Autodesk Fusion 360 part; units mm, degrees
note: some values were not read from the file. Set by a fixed rule: which sketch regions a step uses.
(part 10 of 15)
  line L7918 (197.419, -100.32) -> (197.381, -100.6)
  line L7919 (98.8127, -108.073) -> (99.0879, -108.136)
  line L7920 (197.381, -100.6) -> (197.304, -100.872)
  line L7921 (-22.9133, -112.864) -> (-22.9509, -113.144)
  line L7922 (-23.8113, -111.067) -> (-23.5867, -111.238)
  line L7923 (29.1335, -114.838) -> (28.9254, -114.669)
  line L7924 (-22.9888, -112.181) -> (-22.9293, -112.457)
  line L7925 (29.9879, -111.399) -> (30.2558, -111.384)
  line L7926 (-23.1418, -113.675) -> (-23.2913, -113.914)
  line L7927 (-23.2913, -113.914) -> (-23.4731, -114.13)
  line L7928 (30.2558, -111.384) -> (30.5232, -111.407)
  line L7929 (-23.9184, -114.476) -> (-24.1731, -114.598)
  line L7930 (-23.0276, -113.416) -> (-23.1418, -113.675)
  line L7931 (-22.9509, -113.144) -> (-23.0276, -113.416)
  line L7932 (-24.1731, -114.598) -> (-24.4425, -114.683)
  line L7933 (28.3543, -112.957) -> (28.419, -112.697)
  line L7934 (29.2333, -111.664) -> (29.4714, -111.54)
  line L7935 (29.7246, -111.451) -> (29.9879, -111.399)
  line L7936 (-24.5965, -110.763) -> (-24.3213, -110.827)
  line L7937 (32.0865, -113.669) -> (32.0137, -113.928)
  line L7938 (-24.3213, -110.827) -> (-24.0578, -110.929)
  line L7939 (28.8207, -112.005) -> (29.0149, -111.82)
  line L7940 (-23.4731, -114.13) -> (-23.6835, -114.319)
  line L7941 (-23.3885, -111.44) -> (-23.2207, -111.667)
  line L7942 (-23.6835, -114.319) -> (-23.9184, -114.476)
  line L7943 (-23.5867, -111.238) -> (-23.3885, -111.44)
  line L7944 (-22.9093, -112.739) -> (-22.9133, -112.864)
  line L7945 (29.0149, -111.82) -> (29.2333, -111.664)
  line L7946 (28.3269, -113.224) -> (28.3543, -112.957)
  line L7947 (-23.2207, -111.667) -> (-23.0865, -111.916)
  line L7948 (28.5197, -112.448) -> (28.6545, -112.216)
  line L7949 (29.4714, -111.54) -> (29.7246, -111.451)
  line L7950 (-22.9293, -112.457) -> (-22.9093, -112.739)
  line L7951 (32.1223, -113.403) -> (32.0865, -113.669)
  line L7952 (231.22, -110.094) -> (231.383, -110.183)
  line L7953 (231.643, -110.444) -> (231.73, -110.608)
  line L7954 (96.9389, -111.298) -> (96.7783, -111.066)
  line L7955 (96.8456, -108.924) -> (97.0205, -108.702)
  line L7956 (97.972, -108.119) -> (98.2491, -108.064)
  line L7957 (231.526, -110.301) -> (231.643, -110.444)
  line L7958 (97.0205, -108.702) -> (97.2249, -108.507)
  line L7959 (231.383, -110.183) -> (231.526, -110.301)
  line L7960 (96.5626, -110.545) -> (96.5119, -110.267)
  line L7961 (97.5918, -111.83) -> (97.3498, -111.684)
  line L7962 (97.3498, -111.684) -> (97.1307, -111.506)
  line L7963 (98.2491, -108.064) -> (98.5312, -108.048)
  line L7964 (96.652, -110.813) -> (96.5626, -110.545)
  line L7965 (96.5977, -109.43) -> (96.7037, -109.168)
  line L7966 (97.2249, -108.507) -> (97.4548, -108.343)
  line L7967 (97.1307, -111.506) -> (96.9389, -111.298)
  line L7968 (96.7783, -111.066) -> (96.652, -110.813)
  line L7969 (99.236, -111.908) -> (98.9667, -111.993)
  line L7970 (98.4056, -112.046) -> (98.125, -112.013)
  line L7971 (98.5312, -108.048) -> (98.8127, -108.073)
  line L7972 (97.7055, -108.212) -> (97.972, -108.119)
  line L7973 (97.4548, -108.343) -> (97.7055, -108.212)
  line L7974 (231.778, -111.181) -> (231.72, -111.357)
  line L7975 (231.361, -111.772) -> (231.195, -111.856)
  line L7976 (231.628, -111.518) -> (231.507, -111.658)
  line L7977 (230.332, -110.175) -> (230.496, -110.089)
  line L7978 (229.969, -111.32) -> (229.918, -111.142)
  line L7979 (103.122, -111.801) -> (102.96, -111.71)
  line L7980 (229.902, -110.957) -> (229.923, -110.773)
  line L7981 (230.187, -110.291) -> (230.332, -110.175)
  line L7982 (229.923, -110.773) -> (229.979, -110.596)
  line L7983 (231.802, -110.97) -> (231.802, -110.997)
  line L7984 (230.496, -110.089) -> (230.674, -110.037)
  line L7985 (230.859, -110.02) -> (231.043, -110.04)
  line L7986 (230.832, -111.92) -> (230.648, -111.898)
  line L7987 (230.472, -111.841) -> (230.31, -111.75)
  line L7988 (103.871, -110.054) -> (104.034, -110.143)
  line L7989 (231.017, -111.906) -> (230.832, -111.92)
  line L7990 (230.31, -111.75) -> (230.169, -111.63)
  line L7991 (231.802, -110.997) -> (231.778, -111.181)
  line L7992 (229.979, -110.596) -> (230.068, -110.433)
  line L7993 (103.483, -111.88) -> (103.299, -111.858)
  line L7994 (230.674, -110.037) -> (230.859, -110.02)
  line L7995 (-42.8184, -107.621) -> (-42.5719, -107.759)
  line L7996 (231.72, -111.357) -> (231.628, -111.518)
  line L7997 (230.053, -111.485) -> (229.969, -111.32)
  line L7998 (229.918, -111.142) -> (229.902, -110.957)
  line L7999 (104.034, -110.143) -> (104.177, -110.261)
  line L8000 (231.195, -111.856) -> (231.017, -111.906)
  line L8001 (230.169, -111.63) -> (230.053, -111.485)
  line L8002 (231.784, -110.786) -> (231.802, -110.97)
  line L8003 (230.648, -111.898) -> (230.472, -111.841)
  line L8004 (103.694, -109.999) -> (103.871, -110.054)
  line L8005 (231.73, -110.608) -> (231.784, -110.786)
  line L8006 (104.177, -110.261) -> (104.294, -110.404)
  line L8007 (104.158, -111.618) -> (104.012, -111.732)
  line L8008 (102.982, -110.135) -> (103.147, -110.049)
  line L8009 (104.012, -111.732) -> (103.846, -111.816)
  line L8010 (231.507, -111.658) -> (231.361, -111.772)
  line L8011 (230.068, -110.433) -> (230.187, -110.291)
  line L8012 (102.553, -110.917) -> (102.573, -110.733)
  line L8013 (104.452, -110.957) -> (104.429, -111.141)
  line L8014 (102.629, -110.556) -> (102.719, -110.393)
  line L8015 (102.96, -111.71) -> (102.819, -111.59)
  line L8016 (104.435, -110.746) -> (104.453, -110.93)
  line L8017 (104.37, -111.316) -> (104.279, -111.478)
  line L8018 (102.619, -111.28) -> (102.568, -111.102)
  line L8019 (-43.0818, -107.519) -> (-42.8184, -107.621)
  line L8020 (102.819, -111.59) -> (102.704, -111.445)
  line L8021 (103.147, -110.049) -> (103.325, -109.997)
  line L8022 (102.704, -111.445) -> (102.619, -111.28)
  line L8023 (102.719, -110.393) -> (102.838, -110.251)
  line L8024 (103.509, -109.98) -> (103.694, -109.999)
  line L8025 (104.294, -110.404) -> (104.381, -110.568)
  line L8026 (-42.3473, -107.93) -> (-42.1491, -108.132)
  line L8027 (103.299, -111.858) -> (103.122, -111.801)
  line L8028 (103.668, -111.866) -> (103.483, -111.88)
  line L8029 (103.846, -111.816) -> (103.668, -111.866)
  line L8030 (-42.5719, -107.759) -> (-42.3473, -107.93)
  line L8031 (-42.2337, -110.823) -> (-42.4441, -111.011)
  line L8032 (-41.7493, -108.873) -> (-41.6899, -109.149)
  line L8033 (-45.5177, -110.196) -> (-45.6071, -109.928)
  line L8034 (104.381, -110.568) -> (104.435, -110.746)
  line L8035 (104.453, -110.93) -> (104.452, -110.957)
  line L8036 (102.838, -110.251) -> (102.982, -110.135)
  line L8037 (102.568, -111.102) -> (102.553, -110.917)
  line L8038 (102.573, -110.733) -> (102.629, -110.556)
  line L8039 (-45.6579, -109.65) -> (-45.6689, -109.368)
  line L8040 (-41.7115, -109.836) -> (-41.7882, -110.108)
  line L8041 (103.325, -109.997) -> (103.509, -109.98)
  line L8042 (104.429, -111.141) -> (104.37, -111.316)
  line L8043 (104.279, -111.478) -> (104.158, -111.618)
  line L8044 (-43.3571, -107.455) -> (-43.0818, -107.519)
  line L8045 (-43.4817, -111.422) -> (-43.7641, -111.428)
  line L8046 (-41.7882, -110.108) -> (-41.9024, -110.367)
  line L8047 (-42.679, -111.168) -> (-42.9337, -111.29)
  line L8048 (-43.7641, -111.428) -> (-44.0447, -111.395)
  line L8049 (-45.6401, -109.087) -> (-45.572, -108.813)
  line L8050 (-42.9337, -111.29) -> (-43.203, -111.375)
  line L8051 (-42.1491, -108.132) -> (-41.9813, -108.359)
  line L8052 (-42.0519, -110.606) -> (-42.2337, -110.823)
  line L8053 (-41.9024, -110.367) -> (-42.0519, -110.606)
  line L8054 (-44.0447, -111.395) -> (-44.3178, -111.323)
  line L8055 (-41.6699, -109.431) -> (-41.6739, -109.556)
  line L8056 (-45.3914, -110.449) -> (-45.5177, -110.196)
  line L8057 (-41.6739, -109.556) -> (-41.7115, -109.836)
  line L8058 (-45.2308, -110.681) -> (-45.3914, -110.449)
  line L8059 (-44.5779, -111.213) -> (-44.8199, -111.067)
  line L8060 (-44.8199, -111.067) -> (-45.039, -110.889)
  line L8061 (-45.6071, -109.928) -> (-45.6579, -109.65)
  line L8062 (-45.039, -110.889) -> (-45.2308, -110.681)
  line L8063 (-45.6689, -109.368) -> (-45.6401, -109.087)
  line L8064 (-42.4441, -111.011) -> (-42.679, -111.168)
  line L8065 (-43.203, -111.375) -> (-43.4817, -111.422)
  line L8066 (-37.7992, -110.699) -> (-37.8908, -110.86)
  line L8067 (-37.7171, -110.313) -> (-37.7175, -110.339)
  line L8068 (-38.1581, -111.115) -> (-38.3236, -111.199)
  line L8069 (-43.6385, -107.431) -> (-43.3571, -107.455)
  line L8070 (-45.1492, -108.085) -> (-44.9448, -107.89)
  line L8071 (-37.7175, -110.339) -> (-37.7407, -110.523)
  line L8072 (-38.5021, -111.248) -> (-38.687, -111.263)
  line L8073 (-37.7407, -110.523) -> (-37.7992, -110.699)
  line L8074 (-41.6899, -109.149) -> (-41.6699, -109.431)
  line L8075 (-44.9448, -107.89) -> (-44.7149, -107.725)
  line L8076 (-38.4761, -109.382) -> (-38.299, -109.437)
  line L8077 (-37.993, -109.643) -> (-37.8758, -109.787)
  line L8078 (-41.9813, -108.359) -> (-41.8471, -108.608)
  line L8079 (-38.1359, -109.525) -> (-37.993, -109.643)
  line L8080 (-38.8711, -111.241) -> (-39.0474, -111.183)
  line L8081 (-44.3178, -111.323) -> (-44.5779, -111.213)
  line L8082 (-44.1977, -107.502) -> (-43.9206, -107.446)
  line L8083 (-41.8471, -108.608) -> (-41.7493, -108.873)
  line L8084 (197.423, -100.195) -> (197.419, -100.32)
  line L8085 (196.159, -102.054) -> (195.889, -102.139)
  line L8086 (196.521, -98.5231) -> (196.745, -98.6945)
  line L8087 (195.048, -102.159) -> (194.775, -102.087)
  line L8088 (196.859, -101.587) -> (196.648, -101.775)
  line L8089 (197.304, -100.872) -> (197.19, -101.131)
  line L8090 (196.274, -98.3851) -> (196.521, -98.5231)
  line L8091 (193.701, -101.213) -> (193.575, -100.96)
  line L8092 (194.272, -101.831) -> (194.053, -101.653)
  line L8093 (193.575, -100.96) -> (193.485, -100.692)
  line L8094 (193.435, -100.414) -> (193.423, -100.132)
  line L8095 (193.485, -100.692) -> (193.435, -100.414)
  line L8096 (193.423, -100.132) -> (193.452, -99.8508)
  line L8097 (194.775, -102.087) -> (194.515, -101.977)
  line L8098 (197.041, -101.37) -> (196.859, -101.587)
  line L8099 (196.745, -98.6945) -> (196.943, -98.8958)
  line L8100 (197.343, -99.6367) -> (197.403, -99.9129)
  line L8101 (96.5296, -109.704) -> (96.5977, -109.43)
  line L8102 (197.19, -101.131) -> (197.041, -101.37)
  line L8103 (96.5119, -110.267) -> (96.5008, -109.985)
  line L8104 (96.5008, -109.985) -> (96.5296, -109.704)
  line L8105 (197.245, -99.3717) -> (197.343, -99.6367)
  line L8106 (196.648, -101.775) -> (196.413, -101.932)
  line L8107 (194.515, -101.977) -> (194.272, -101.831)
  line L8108 (99.4907, -111.785) -> (99.236, -111.908)
  line L8109 (98.125, -112.013) -> (97.852, -111.94)
  line L8110 (194.053, -101.653) -> (193.862, -101.445)
  line L8111 (97.852, -111.94) -> (97.5918, -111.83)
  line L8112 (231.043, -110.04) -> (231.22, -110.094)
  line L8113 (98.688, -112.039) -> (98.4056, -112.046)
  line L8114 (196.413, -101.932) -> (196.159, -102.054)
  line L8115 (96.7037, -109.168) -> (96.8456, -108.924)
  line L8116 (98.9667, -111.993) -> (98.688, -112.039)
  line L8117 (262.602, -142.986) -> (262.452, -143.226)
  line L8118 (262.716, -142.727) -> (262.602, -142.986)
  line L8119 (247.27, -147.655) -> (247.093, -147.598)
  line L8120 (262.355, -140.751) -> (262.523, -140.978)
  line L8121 (247.093, -147.598) -> (246.931, -147.507)
  line L8122 (262.157, -140.55) -> (262.355, -140.751)
  line L8123 (246.953, -145.932) -> (247.118, -145.846)
  line L8124 (262.452, -143.226) -> (262.271, -143.442)
  line L8125 (247.296, -145.794) -> (247.48, -145.777)
  line L8126 (246.79, -147.387) -> (246.675, -147.242)
  line L8127 (262.793, -142.456) -> (262.716, -142.727)
  line L8128 (261.422, -140.138) -> (261.686, -140.24)
  line L8129 (247.118, -145.846) -> (247.296, -145.794)
  line L8130 (261.686, -140.24) -> (261.932, -140.378)
  line L8131 (246.931, -147.507) -> (246.79, -147.387)
  line L8132 (246.544, -146.53) -> (246.6, -146.353)
  line L8133 (246.675, -147.242) -> (246.59, -147.077)
  line L8134 (142.059, -170.379) -> (142.008, -170.201)
  line L8135 (246.59, -147.077) -> (246.539, -146.899)
  line L8136 (246.6, -146.353) -> (246.69, -146.19)
  line L8137 (262.657, -141.227) -> (262.755, -141.492)
  line L8138 (191.042, -169.597) -> (191.186, -169.481)
  line L8139 (143.451, -170.831) -> (143.286, -170.915)
  line L8140 (143.821, -169.667) -> (143.874, -169.845)
  line L8141 (143.733, -169.504) -> (143.821, -169.667)
  line L8142 (141.992, -170.016) -> (142.013, -169.832)
  line L8143 (143.874, -169.845) -> (143.892, -170.029)
  line L8144 (142.764, -169.096) -> (142.949, -169.079)
  line L8145 (142.949, -169.079) -> (143.133, -169.099)
  line L8146 (247.48, -145.777) -> (247.665, -145.796)
  line L8147 (190.923, -169.739) -> (191.042, -169.597)
  line L8148 (246.539, -146.899) -> (246.524, -146.714)
  line L8149 (191.186, -169.481) -> (191.351, -169.395)
  line L8150 (190.833, -169.901) -> (190.923, -169.739)
  line L8151 (191.351, -169.395) -> (191.529, -169.342)
  line L8152 (262.83, -142.176) -> (262.793, -142.456)
  line L8153 (196.899, -166.217) -> (197.162, -166.319)
  line L8154 (143.133, -169.099) -> (143.31, -169.154)
  line L8155 (261.147, -140.075) -> (261.422, -140.138)
  line L8156 (190.777, -170.078) -> (190.833, -169.901)
  line L8157 (142.738, -170.957) -> (142.562, -170.9)
  line L8158 (191.713, -169.325) -> (191.898, -169.345)
  line L8159 (142.013, -169.832) -> (142.069, -169.655)
  line L8160 (142.158, -169.493) -> (142.278, -169.351)
  line L8161 (191.529, -169.342) -> (191.713, -169.325)
  line L8162 (246.809, -146.048) -> (246.953, -145.932)
  line L8163 (262.523, -140.978) -> (262.657, -141.227)
  line L8164 (143.473, -169.242) -> (143.616, -169.36)
  line L8165 (143.892, -170.029) -> (143.892, -170.056)
  line L8166 (190.757, -170.262) -> (190.777, -170.078)
  line L8167 (246.69, -146.19) -> (246.809, -146.048)
  line L8168 (261.932, -140.378) -> (262.157, -140.55)
  line L8169 (246.524, -146.714) -> (246.544, -146.53)
  line L8170 (142.144, -170.544) -> (142.059, -170.379)
  line L8171 (143.31, -169.154) -> (143.473, -169.242)
  line L8172 (142.278, -169.351) -> (142.422, -169.234)
  line L8173 (262.834, -142.05) -> (262.83, -142.176)
  line L8174 (262.814, -141.768) -> (262.834, -142.05)
  line L8175 (142.069, -169.655) -> (142.158, -169.493)
  line L8176 (262.755, -141.492) -> (262.814, -141.768)
  line L8177 (143.869, -170.24) -> (143.81, -170.416)
  line L8178 (196.216, -170.126) -> (195.936, -170.093)
  line L8179 (195.161, -169.765) -> (194.941, -169.586)
  line L8180 (143.892, -170.056) -> (143.869, -170.24)
  line L8181 (142.259, -170.689) -> (142.144, -170.544)
  line L8182 (142.008, -170.201) -> (141.992, -170.016)
  line L8183 (198.311, -168.129) -> (198.307, -168.254)
  line L8184 (196.777, -170.073) -> (196.499, -170.12)
  line L8185 (197.999, -167.057) -> (198.133, -167.306)
  line L8186 (142.422, -169.234) -> (142.586, -169.149)
  line L8187 (197.633, -166.628) -> (197.831, -166.83)
  line L8188 (197.536, -169.709) -> (197.302, -169.866)
  line L8189 (139.661, -166.382) -> (139.859, -166.584)
  line L8190 (198.078, -169.064) -> (197.929, -169.304)
  line L8191 (196.623, -166.153) -> (196.899, -166.217)
  line L8192 (194.589, -169.147) -> (194.463, -168.894)
  line L8193 (197.409, -166.457) -> (197.633, -166.628)
  line L8194 (139.859, -166.584) -> (140.027, -166.811)
  line L8195 (198.231, -167.571) -> (198.291, -167.847)
  line L8196 (142.586, -169.149) -> (142.764, -169.096)
  line L8197 (197.162, -166.319) -> (197.409, -166.457)
  line L8198 (197.747, -169.52) -> (197.536, -169.709)
  line L8199 (140.318, -167.601) -> (140.338, -167.882)
  line L8200 (194.656, -167.004) -> (194.831, -166.783)
  line L8201 (194.312, -168.066) -> (194.34, -167.785)
  line L8202 (194.831, -166.783) -> (195.036, -166.588)
  line L8203 (197.831, -166.83) -> (197.999, -167.057)
  line L8204 (198.291, -167.847) -> (198.311, -168.129)
  line L8205 (195.266, -166.423) -> (195.516, -166.293)
  line L8206 (142.922, -170.979) -> (142.738, -170.957)
  line L8207 (194.75, -169.379) -> (194.589, -169.147)
  line L8208 (143.81, -170.416) -> (143.719, -170.577)
  line L8209 (197.302, -169.866) -> (197.047, -169.988)
  line L8210 (195.663, -170.021) -> (195.403, -169.911)
  line L8211 (140.338, -167.882) -> (140.334, -168.008)
  line L8212 (143.107, -170.965) -> (142.922, -170.979)
  line L8213 (142.562, -170.9) -> (142.4, -170.809)
  line L8214 (143.286, -170.915) -> (143.107, -170.965)
  line L8215 (143.719, -170.577) -> (143.597, -170.717)
  line L8216 (198.269, -168.534) -> (198.192, -168.806)
  line L8217 (195.936, -170.093) -> (195.663, -170.021)
  line L8218 (198.307, -168.254) -> (198.269, -168.534)
  line L8219 (194.941, -169.586) -> (194.75, -169.379)
  line L8220 (143.597, -170.717) -> (143.451, -170.831)
  line L8221 (194.373, -168.626) -> (194.323, -168.348)
  line L8222 (194.323, -168.348) -> (194.312, -168.066)
  line L8223 (197.929, -169.304) -> (197.747, -169.52)
  line L8224 (197.047, -169.988) -> (196.777, -170.073)
  line L8225 (143.616, -169.36) -> (143.733, -169.504)
  line L8226 (198.133, -167.306) -> (198.231, -167.571)
  line L8227 (198.192, -168.806) -> (198.078, -169.064)
  line L8228 (194.463, -168.894) -> (194.373, -168.626)
  line L8229 (142.4, -170.809) -> (142.259, -170.689)
  line L8230 (195.403, -169.911) -> (195.161, -169.765)
  line L8231 (196.499, -170.12) -> (196.216, -170.126)
  line L8232 (137.188, -169.519) -> (136.969, -169.34)
  line L8233 (140.027, -166.811) -> (140.161, -167.059)
  line L8234 (138.526, -169.874) -> (138.244, -169.88)
  line L8235 (140.297, -168.288) -> (140.22, -168.56)
  line L8236 (138.244, -169.88) -> (137.963, -169.847)
  line L8237 (139.564, -169.463) -> (139.329, -169.62)
  line L8238 (196.06, -166.144) -> (196.342, -166.129)
  line L8239 (137.43, -169.664) -> (137.188, -169.519)
  line L8240 (139.074, -169.742) -> (138.805, -169.827)
  line L8241 (194.408, -167.511) -> (194.515, -167.249)
  line L8242 (136.436, -167.264) -> (136.542, -167.003)
  line L8243 (201.283, -165.106) -> (201.446, -165.194)
  line L8244 (201.793, -165.62) -> (201.847, -165.797)
  line L8245 (195.783, -166.199) -> (196.06, -166.144)
  line L8246 (136.49, -168.648) -> (136.401, -168.38)
  line L8247 (201.106, -165.051) -> (201.283, -165.106)
  line L8248 (201.847, -165.797) -> (201.865, -165.982)
  line L8249 (137.81, -165.953) -> (138.088, -165.898)
  line L8250 (138.651, -165.907) -> (138.926, -165.971)
  line L8251 (195.036, -166.588) -> (195.266, -166.423)
  line L8252 (140.22, -168.56) -> (140.106, -168.818)
  line L8253 (194.515, -167.249) -> (194.656, -167.004)
  line L8254 (137.69, -169.775) -> (137.43, -169.664)
  line L8255 (137.293, -166.177) -> (137.544, -166.047)
  line L8256 (139.19, -166.073) -> (139.436, -166.211)
  line L8257 (138.088, -165.898) -> (138.37, -165.883)
  line L8258 (137.963, -169.847) -> (137.69, -169.775)
  line L8259 (200.041, -165.607) -> (200.131, -165.445)
  line L8260 (137.063, -166.341) -> (137.293, -166.177)
  line L8261 (200.737, -165.048) -> (200.921, -165.032)
  line L8262 (136.777, -169.133) -> (136.617, -168.901)
  line L8263 (139.956, -169.058) -> (139.774, -169.274)
  line L8264 (200.559, -165.101) -> (200.737, -165.048)
  line L8265 (201.691, -166.529) -> (201.57, -166.67)
  line L8266 (136.339, -167.82) -> (136.368, -167.539)
  line L8267 (200.895, -166.931) -> (200.711, -166.909)
  line L8268 (200.031, -166.331) -> (199.98, -166.153)
  line L8269 (140.106, -168.818) -> (139.956, -169.058)
  line L8270 (195.516, -166.293) -> (195.783, -166.199)
  line L8271 (139.436, -166.211) -> (139.661, -166.382)
  line L8272 (140.259, -167.324) -> (140.318, -167.601)
  line L8273 (138.926, -165.971) -> (139.19, -166.073)
  line L8274 (136.401, -168.38) -> (136.35, -168.102)
  line L8275 (138.805, -169.827) -> (138.526, -169.874)
  line L8276 (139.774, -169.274) -> (139.564, -169.463)
  line L8277 (136.859, -166.536) -> (137.063, -166.341)
  line L8278 (140.161, -167.059) -> (140.259, -167.324)
  line L8279 (139.329, -169.62) -> (139.074, -169.742)
  line L8280 (201.446, -165.194) -> (201.589, -165.312)
  line L8281 (140.334, -168.008) -> (140.297, -168.288)
  line L8282 (201.589, -165.312) -> (201.706, -165.456)
  line L8283 (201.706, -165.456) -> (201.793, -165.62)
  line L8284 (138.37, -165.883) -> (138.651, -165.907)
  line L8285 (136.542, -167.003) -> (136.684, -166.758)
  line L8286 (201.865, -165.982) -> (201.864, -166.008)
  line L8287 (136.969, -169.34) -> (136.777, -169.133)
  line L8288 (194.34, -167.785) -> (194.408, -167.511)
  line L8289 (136.617, -168.901) -> (136.49, -168.648)
  line L8290 (136.368, -167.539) -> (136.436, -167.264)
  line L8291 (136.35, -168.102) -> (136.339, -167.82)
  line L8292 (196.342, -166.129) -> (196.623, -166.153)
  line L8293 (136.684, -166.758) -> (136.859, -166.536)
  line L8294 (137.544, -166.047) -> (137.81, -165.953)
  line L8295 (201.08, -166.917) -> (200.895, -166.931)
  line L8296 (134.612, -165.374) -> (134.666, -165.551)
  line L8297 (200.25, -165.303) -> (200.394, -165.187)
  line L8298 (200.534, -166.852) -> (200.372, -166.762)
  line L8299 (201.424, -166.784) -> (201.258, -166.867)
  line L8300 (200.131, -165.445) -> (200.25, -165.303)
  line L8301 (200.921, -165.032) -> (201.106, -165.051)
  line L8302 (134.408, -165.066) -> (134.525, -165.21)
  line L8303 (201.57, -166.67) -> (201.424, -166.784)
  line L8304 (200.231, -166.642) -> (200.116, -166.496)
  line L8305 (200.711, -166.909) -> (200.534, -166.852)
  line L8306 (201.864, -166.008) -> (201.841, -166.192)
  line L8307 (199.98, -166.153) -> (199.965, -165.968)
  line L8308 (134.525, -165.21) -> (134.612, -165.374)
  line L8309 (200.394, -165.187) -> (200.559, -165.101)
  line L8310 (200.116, -166.496) -> (200.031, -166.331)
  line L8311 (134.666, -165.551) -> (134.684, -165.736)
  line L8312 (201.841, -166.192) -> (201.782, -166.368)
  line L8313 (201.258, -166.867) -> (201.08, -166.917)
  line L8314 (133.925, -164.805) -> (134.102, -164.86)
  line L8315 (134.265, -164.948) -> (134.408, -165.066)
  line L8316 (199.965, -165.968) -> (199.985, -165.784)
  line L8317 (201.782, -166.368) -> (201.691, -166.529)
  line L8318 (133.53, -166.663) -> (133.354, -166.606)
  line L8319 (133.354, -166.606) -> (133.192, -166.516)
  line L8320 (132.8, -165.907) -> (132.784, -165.722)
  line L8321 (132.861, -165.361) -> (132.95, -165.199)
  line L8322 (134.243, -166.538) -> (134.078, -166.621)
  line L8323 (200.372, -166.762) -> (200.231, -166.642)
  line L8324 (214.16, -159.888) -> (214.213, -160.065)
  line L8325 (213.813, -159.462) -> (213.956, -159.58)
  line L8326 (132.784, -165.722) -> (132.805, -165.538)
  line L8327 (134.078, -166.621) -> (133.899, -166.671)
  line L8328 (132.936, -166.25) -> (132.851, -166.085)
  line L8329 (133.214, -164.941) -> (133.378, -164.855)
  line L8330 (133.378, -164.855) -> (133.556, -164.802)
  line L8331 (134.102, -164.86) -> (134.265, -164.948)
  line L8332 (213.956, -159.58) -> (214.073, -159.724)
  line L8333 (214.073, -159.724) -> (214.16, -159.888)
  line L8334 (132.95, -165.199) -> (133.069, -165.057)
  line L8335 (134.684, -165.736) -> (134.684, -165.762)
  line L8336 (133.899, -166.671) -> (133.714, -166.685)
  line L8337 (213.65, -159.374) -> (213.813, -159.462)
  line L8338 (199.985, -165.784) -> (200.041, -165.607)
  line L8339 (134.661, -165.946) -> (134.602, -166.122)
  line L8340 (132.805, -165.538) -> (132.861, -165.361)
  line L8341 (133.192, -166.516) -> (133.051, -166.395)
  line L8342 (134.684, -165.762) -> (134.661, -165.946)
  line L8343 (133.714, -166.685) -> (133.53, -166.663)
  line L8344 (134.51, -166.283) -> (134.389, -166.424)
  line L8345 (133.069, -165.057) -> (133.214, -164.941)
  line L8346 (133.556, -164.802) -> (133.741, -164.786)
  line L8347 (134.602, -166.122) -> (134.51, -166.283)
  line L8348 (133.051, -166.395) -> (132.936, -166.25)
  line L8349 (213.473, -159.319) -> (213.65, -159.374)
  line L8350 (132.851, -166.085) -> (132.8, -165.907)
  line L8351 (133.741, -164.786) -> (133.925, -164.805)
  line L8352 (213.447, -161.185) -> (213.262, -161.199)
  line L8353 (212.739, -161.03) -> (212.598, -160.909)
  line L8354 (212.398, -160.599) -> (212.347, -160.421)
  line L8355 (214.149, -160.636) -> (214.058, -160.797)
  line L8356 (212.483, -160.764) -> (212.398, -160.599)
  line L8357 (212.926, -159.369) -> (213.104, -159.316)
  line L8358 (214.231, -160.276) -> (214.208, -160.46)
  line L8359 (212.352, -160.052) -> (212.408, -159.875)
  line L8360 (213.078, -161.177) -> (212.901, -161.12)
  line L8361 (214.213, -160.065) -> (214.232, -160.25)
  line L8362 (213.625, -161.135) -> (213.447, -161.185)
  line L8363 (212.901, -161.12) -> (212.739, -161.03)
  line L8364 (121.769, -159.225) -> (121.912, -159.343)
  line L8365 (212.598, -160.909) -> (212.483, -160.764)
  line L8366 (121.912, -159.343) -> (122.029, -159.487)
  line L8367 (121.606, -159.136) -> (121.769, -159.225)
  line L8368 (213.104, -159.316) -> (213.288, -159.3)
  line L8369 (122.029, -159.487) -> (122.116, -159.65)
  line L8370 (214.208, -160.46) -> (214.149, -160.636)
  line L8371 (134.389, -166.424) -> (134.243, -166.538)
  line L8372 (214.058, -160.797) -> (213.937, -160.938)
  line L8373 (213.288, -159.3) -> (213.473, -159.319)
  line L8374 (212.408, -159.875) -> (212.498, -159.713)
  line L8375 (121.429, -159.082) -> (121.606, -159.136)
  line L8376 (213.791, -161.052) -> (213.625, -161.135)
  line L8377 (212.347, -160.421) -> (212.332, -160.236)
  line L8378 (212.761, -159.455) -> (212.926, -159.369)
  line L8379 (212.617, -159.571) -> (212.761, -159.455)
  line L8380 (214.232, -160.25) -> (214.231, -160.276)
  line L8381 (213.937, -160.938) -> (213.791, -161.052)
  line L8382 (122.188, -160.012) -> (122.188, -160.039)
  line L8383 (120.573, -159.334) -> (120.718, -159.217)
  line L8384 (212.332, -160.236) -> (212.352, -160.052)
  line L8385 (212.498, -159.713) -> (212.617, -159.571)
  line L8386 (122.188, -160.039) -> (122.164, -160.223)
  line L8387 (122.164, -160.223) -> (122.106, -160.399)
  line L8388 (121.581, -160.898) -> (121.403, -160.948)
  line L8389 (218.474, -156.191) -> (218.737, -156.293)
  line L8390 (120.309, -159.815) -> (120.365, -159.638)
  line L8391 (121.403, -160.948) -> (121.218, -160.962)
  line L8392 (121.245, -159.062) -> (121.429, -159.082)
  line L8393 (120.288, -159.999) -> (120.309, -159.815)
  line L8394 (213.262, -161.199) -> (213.078, -161.177)
  line L8395 (218.737, -156.293) -> (218.984, -156.431)
  line L8396 (120.718, -159.217) -> (120.882, -159.131)
  line L8397 (120.454, -159.476) -> (120.573, -159.334)
  line L8398 (122.17, -159.828) -> (122.188, -160.012)
  line L8399 (121.747, -160.814) -> (121.581, -160.898)
  line L8400 (121.893, -160.7) -> (121.747, -160.814)
  line L8401 (122.116, -159.65) -> (122.17, -159.828)
  line L8402 (122.014, -160.56) -> (121.893, -160.7)
  line L8403 (121.218, -160.962) -> (121.034, -160.94)
  line L8404 (120.355, -160.362) -> (120.304, -160.184)
  line L8405 (218.984, -156.431) -> (219.208, -156.602)
  line L8406 (120.439, -160.527) -> (120.355, -160.362)
  line L8407 (120.882, -159.131) -> (121.06, -159.079)
  line L8408 (121.034, -160.94) -> (120.858, -160.883)
  line L8409 (120.858, -160.883) -> (120.696, -160.792)
  line L8410 (120.696, -160.792) -> (120.555, -160.672)
  line L8411 (121.06, -159.079) -> (121.245, -159.062)
  line L8412 (122.106, -160.399) -> (122.014, -160.56)
  line L8413 (120.555, -160.672) -> (120.439, -160.527)
  line L8414 (219.866, -157.821) -> (219.886, -158.103)
  line L8415 (219.882, -158.228) -> (219.844, -158.508)
  line L8416 (216.164, -159.121) -> (216.038, -158.868)
  line L8417 (219.886, -158.103) -> (219.882, -158.228)
  line L8418 (216.517, -159.561) -> (216.325, -159.353)
  line L8419 (216.325, -159.353) -> (216.164, -159.121)
  line L8420 (218.353, -160.047) -> (218.074, -160.094)
  line L8421 (216.038, -158.868) -> (215.948, -158.6)
  line L8422 (215.948, -158.6) -> (215.898, -158.322)
  line L8423 (219.574, -157.031) -> (219.708, -157.28)
  line L8424 (219.504, -159.278) -> (219.322, -159.494)
  line L8425 (219.322, -159.494) -> (219.111, -159.683)
  line L8426 (120.365, -159.638) -> (120.454, -159.476)
  line L8427 (120.304, -160.184) -> (120.288, -159.999)
  line L8428 (218.198, -156.127) -> (218.474, -156.191)
  line L8429 (219.208, -156.602) -> (219.406, -156.804)
  line L8430 (216.736, -159.739) -> (216.517, -159.561)
  line L8431 (219.708, -157.28) -> (219.806, -157.545)
  line L8432 (218.622, -159.962) -> (218.353, -160.047)
  line L8433 (217.238, -159.995) -> (216.978, -159.885)
  line L8434 (218.074, -160.094) -> (217.791, -160.1)
  line L8435 (216.978, -159.885) -> (216.736, -159.739)
  line L8436 (219.806, -157.545) -> (219.866, -157.821)
  line L8437 (219.406, -156.804) -> (219.574, -157.031)
  line L8438 (217.791, -160.1) -> (217.511, -160.067)
  line L8439 (215.898, -158.322) -> (215.887, -158.04)
  line L8440 (215.887, -158.04) -> (215.915, -157.759)
  line L8441 (215.915, -157.759) -> (215.984, -157.485)
  line L8442 (215.984, -157.485) -> (216.09, -157.223)
  line L8443 (219.767, -158.78) -> (219.653, -159.039)
  line L8444 (219.653, -159.039) -> (219.504, -159.278)
  line L8445 (219.844, -158.508) -> (219.767, -158.78)
  line L8446 (217.511, -160.067) -> (217.238, -159.995)
  line L8447 (219.111, -159.683) -> (218.877, -159.84)
  line L8448 (218.877, -159.84) -> (218.622, -159.962)
  line L8449 (118.252, -159.041) -> (118.07, -159.257)
  line L8450 (216.406, -156.757) -> (216.611, -156.562)
  line L8451 (117.485, -156.056) -> (117.732, -156.194)
  line L8452 (217.091, -156.267) -> (217.358, -156.174)
  line L8453 (116.947, -155.89) -> (117.222, -155.954)
  line L8454 (117.86, -159.446) -> (117.625, -159.603)
  line L8455 (217.917, -156.103) -> (218.198, -156.127)
  line L8456 (118.614, -157.584) -> (118.634, -157.865)
  line L8457 (117.101, -159.81) -> (116.822, -159.856)
  line L8458 (216.841, -156.397) -> (217.091, -156.267)
  line L8459 (117.625, -159.603) -> (117.37, -159.725)
  line L8460 (118.554, -157.307) -> (118.614, -157.584)
  line L8461 (118.457, -157.042) -> (118.554, -157.307)
  line L8462 (118.634, -157.865) -> (118.63, -157.991)
  line L8463 (118.07, -159.257) -> (117.86, -159.446)
  line L8464 (118.323, -156.794) -> (118.457, -157.042)
  line L8465 (216.231, -156.979) -> (216.406, -156.757)
  line L8466 (116.822, -159.856) -> (116.54, -159.863)
  line L8467 (116.54, -159.863) -> (116.259, -159.83)
  line L8468 (118.63, -157.991) -> (118.592, -158.271)
  line L8469 (117.957, -156.365) -> (118.155, -156.566)
  line L8470 (118.155, -156.566) -> (118.323, -156.794)
  line L8471 (216.611, -156.562) -> (216.841, -156.397)
  line L8472 (117.732, -156.194) -> (117.957, -156.365)
  line L8473 (118.592, -158.271) -> (118.516, -158.543)
  line L8474 (118.516, -158.543) -> (118.401, -158.801)
  line L8475 (118.401, -158.801) -> (118.252, -159.041)
  line L8476 (216.09, -157.223) -> (216.231, -156.979)
  line L8477 (114.635, -157.803) -> (114.664, -157.522)
  line L8478 (115.84, -156.03) -> (116.106, -155.936)
  line L8479 (115.726, -159.647) -> (115.484, -159.502)
  line L8480 (115.073, -159.116) -> (114.912, -158.883)
  line L8481 (117.222, -155.954) -> (117.485, -156.056)
  line L8482 (114.664, -157.522) -> (114.732, -157.247)
  line L8483 (114.732, -157.247) -> (114.838, -156.985)
  line L8484 (115.986, -159.758) -> (115.726, -159.647)
  line L8485 (117.37, -159.725) -> (117.101, -159.81)
  line L8486 (217.358, -156.174) -> (217.635, -156.118)
  line L8487 (217.635, -156.118) -> (217.917, -156.103)
  line L8488 (-38.9911, -72.4069) -> (-39.0419, -72.129)
  line L8489 (-37.8482, -70.074) -> (-37.5817, -69.9804)
  line L8490 (-31.1247, -73.0021) -> (-31.1832, -73.178)
  line L8491 (-36.8657, -73.9006) -> (-37.1481, -73.9073)
  line L8492 (176.301, -71.8785) -> (176.403, -72.0184)
  line L8493 (-39.0242, -71.5656) -> (-38.956, -71.2915)
  line L8494 (-32.7158, -72.1129) -> (-32.5713, -71.9967)
  line L8495 (-31.2598, -72.2659) -> (-31.1728, -72.4296)
  line L8496 (-32.9243, -72.4174) -> (-32.835, -72.2549)
  line L8497 (-31.1192, -72.6071) -> (-31.1011, -72.7916)
  line L8498 (-31.8601, -71.861) -> (-31.683, -71.9159)
  line L8499 (176.013, -71.687) -> (176.168, -71.766)
  line L8500 (-35.2864, -72.8454) -> (-35.4359, -73.0851)
  line L8501 (-38.7754, -72.9276) -> (-38.9017, -72.6749)
  line L8502 (-38.6148, -73.16) -> (-38.7754, -72.9276)
  line L8503 (-31.7076, -73.6773) -> (-31.8861, -73.7272)
  line L8504 (-31.8861, -73.7272) -> (-32.071, -73.7414)
  line L8505 (-35.0579, -72.0351) -> (-35.0955, -72.3151)
  line L8506 (-38.85, -71.0296) -> (-38.7081, -70.7853)
  line L8507 (-36.7411, -69.9341) -> (-36.4659, -69.9979)
  line L8508 (-37.3046, -69.9253) -> (-37.0225, -69.9097)
  line L8509 (-37.0225, -69.9097) -> (-36.7411, -69.9341)
  line L8510 (-38.7081, -70.7853) -> (-38.5332, -70.5635)
  line L8511 (-36.3177, -73.7691) -> (-36.587, -73.8542)
  line L8512 (-31.1011, -72.7916) -> (-31.1015, -72.8182)
  line L8513 (-38.423, -73.3674) -> (-38.6148, -73.16)
  line L8514 (-37.9619, -73.6915) -> (-38.2039, -73.5458)
  line L8515 (-38.0989, -70.2042) -> (-37.8482, -70.074)
  line L8516 (-31.2748, -73.3392) -> (-31.396, -73.4796)
  line L8517 (-36.587, -73.8542) -> (-36.8657, -73.9006)
  line L8518 (-32.5933, -73.5717) -> (-32.7345, -73.4516)
  line L8519 (109.763, -72.5281) -> (109.941, -72.4757)
  line L8520 (-31.683, -71.9159) -> (-31.5199, -72.004)
  line L8521 (-36.063, -73.6468) -> (-36.3177, -73.7691)
  line L8522 (-39.0529, -71.8467) -> (-39.0242, -71.5656)
  line L8523 (-32.9804, -72.5941) -> (-32.9243, -72.4174)
  line L8524 (-32.2291, -71.8585) -> (-32.0445, -71.8417)
  line L8525 (-38.956, -71.2915) -> (-38.85, -71.0296)
  line L8526 (110.125, -72.4589) -> (110.31, -72.4783)
  line L8527 (109.598, -72.614) -> (109.763, -72.5281)
  line L8528 (-38.2039, -73.5458) -> (-38.423, -73.3674)
  line L8529 (-39.0419, -72.129) -> (-39.0529, -71.8467)
  line L8530 (175.845, -71.6458) -> (176.013, -71.687)
  line L8531 (-31.377, -72.1222) -> (-31.2598, -72.2659)
  line L8532 (-37.7018, -73.8017) -> (-37.9619, -73.6915)
  line L8533 (-32.9855, -72.9631) -> (-33.001, -72.7784)
  line L8534 (-32.7345, -73.4516) -> (-32.8497, -73.3063)
  line L8535 (-37.1481, -73.9073) -> (-37.4287, -73.8741)
  line L8536 (-32.5713, -71.9967) -> (-32.407, -71.9108)
  line L8537 (-31.5199, -72.004) -> (-31.377, -72.1222)
  line L8538 (-31.1728, -72.4296) -> (-31.1192, -72.6071)
  line L8539 (-31.1832, -73.178) -> (-31.2748, -73.3392)
  line L8540 (-35.1333, -71.3515) -> (-35.0739, -71.6277)
  line L8541 (-36.2024, -70.0998) -> (-35.9559, -70.2379)
  line L8542 (-36.4659, -69.9979) -> (-36.2024, -70.0998)
  line L8543 (109.184, -73.5804) -> (109.169, -73.3957)
  line L8544 (-35.3653, -70.8378) -> (-35.2311, -71.0865)
  line L8545 (-38.5332, -70.5635) -> (-38.3288, -70.3685)
  line L8546 (-37.4287, -73.8741) -> (-37.7018, -73.8017)
  line L8547 (-37.5817, -69.9804) -> (-37.3046, -69.9253)
  line L8548 (109.941, -72.4757) -> (110.125, -72.4589)
  line L8549 (-38.3288, -70.3685) -> (-38.0989, -70.2042)
  line L8550 (-35.1722, -72.587) -> (-35.2864, -72.8454)
  line L8551 (-38.9017, -72.6749) -> (-38.9911, -72.4069)
  line L8552 (160.25, -72.5228) -> (160.2, -72.6891)
  line L8553 (-32.835, -72.2549) -> (-32.7158, -72.1129)
  line L8554 (174.271, -71.8146) -> (174.416, -71.7194)
  line L8555 (160.2, -72.6891) -> (160.113, -72.8393)
  line L8556 (174.579, -71.6601) -> (174.752, -71.64)
  line L8557 (176.233, -72.9654) -> (176.088, -73.0606)
  line L8558 (160.261, -72.3494) -> (160.25, -72.5228)
  line L8559 (174.203, -72.9015) -> (174.101, -72.7616)
  line L8560 (176.353, -72.8393) -> (176.233, -72.9654)
  line L8561 (174.659, -73.1342) -> (174.491, -73.093)
  line L8562 (-32.4314, -73.6622) -> (-32.5933, -73.5717)
  line L8563 (174.752, -71.64) -> (175.752, -71.64)
  line L8564 (175.752, -73.14) -> (174.752, -73.14)
  line L8565 (176.471, -72.1782) -> (176.501, -72.3494)
  line L8566 (174.064, -72.0909) -> (174.151, -71.9407)
  line L8567 (176.088, -73.0606) -> (175.925, -73.1199)
  line L8568 (176.49, -72.5228) -> (176.44, -72.6891)
  line L8569 (-32.407, -71.9108) -> (-32.2291, -71.8585)
  line L8570 (174.752, -73.14) -> (174.659, -73.1342)
  line L8571 (174.151, -71.9407) -> (174.271, -71.8146)
  line L8572 (174.014, -72.2572) -> (174.064, -72.0909)
  line L8573 (160.163, -72.0184) -> (160.231, -72.1782)
  line L8574 (174.416, -71.7194) -> (174.579, -71.6601)
  line L8575 (157.774, -72.2572) -> (157.824, -72.0909)
  line L8576 (158.512, -71.64) -> (159.512, -71.64)
  line L8577 (175.925, -73.1199) -> (175.752, -73.14)
  line L8578 (234.61, -70.8089) -> (234.773, -70.8971)
  line L8579 (158.031, -71.8146) -> (158.176, -71.7194)
  line L8580 (-33.001, -72.7784) -> (-32.9804, -72.5941)
  line L8581 (159.685, -73.1199) -> (159.512, -73.14)
  line L8582 (234.433, -70.7541) -> (234.61, -70.8089)
  line L8583 (176.501, -72.3494) -> (176.49, -72.5228)
  line L8584 (157.824, -72.0909) -> (157.911, -71.9407)
  line L8585 (158.176, -71.7194) -> (158.339, -71.6601)
  line L8586 (235.173, -71.5002) -> (235.192, -71.6847)
  line L8587 (174.033, -72.6018) -> (174.003, -72.4306)
  line L8588 (175.752, -71.64) -> (175.845, -71.6458)
  line L8589 (160.231, -72.1782) -> (160.261, -72.3494)
  line L8590 (176.44, -72.6891) -> (176.353, -72.8393)
  line L8591 (-32.2551, -73.7195) -> (-32.4314, -73.6622)
  line L8592 (159.605, -71.6458) -> (159.773, -71.687)
  line L8593 (174.101, -72.7616) -> (174.033, -72.6018)
  line L8594 (174.491, -73.093) -> (174.336, -73.014)
  line L8595 (235.192, -71.6847) -> (235.191, -71.7112)
  line L8596 (-32.8497, -73.3063) -> (-32.9344, -73.1414)
  line L8597 (159.928, -71.766) -> (160.061, -71.8785)
  line L8598 (-31.396, -73.4796) -> (-31.5421, -73.5937)
  line L8599 (174.003, -72.4306) -> (174.014, -72.2572)
  line L8600 (174.336, -73.014) -> (174.203, -72.9015)
  line L8601 (234.916, -71.0153) -> (235.033, -71.159)
  line L8602 (157.793, -72.6018) -> (157.763, -72.4306)
  line L8603 (158.251, -73.093) -> (158.096, -73.014)
  line L8604 (159.848, -73.0606) -> (159.685, -73.1199)
  line L8605 (160.061, -71.8785) -> (160.163, -72.0184)
  line L8606 (158.096, -73.014) -> (157.963, -72.9015)
  line L8607 (235.191, -71.7112) -> (235.168, -71.8952)
  line L8608 (-31.1015, -72.8182) -> (-31.1247, -73.0021)
  line L8609 (176.168, -71.766) -> (176.301, -71.8785)
  line L8610 (-32.071, -73.7414) -> (-32.2551, -73.7195)
  line L8611 (-32.9344, -73.1414) -> (-32.9855, -72.9631)
  line L8612 (176.403, -72.0184) -> (176.471, -72.1782)
  line L8613 (159.773, -71.687) -> (159.928, -71.766)
  line L8614 (-31.5421, -73.5937) -> (-31.7076, -73.6773)
  line L8615 (-32.0445, -71.8417) -> (-31.8601, -71.861)
  line L8616 (234.751, -72.4868) -> (234.585, -72.5704)
  line L8617 (158.419, -73.1342) -> (158.251, -73.093)
  line L8618 (101.063, -71.6447) -> (101.063, -71.6712)
  line L8619 (234.064, -70.7515) -> (234.248, -70.7347)
  line L8620 (235.033, -71.159) -> (235.12, -71.3227)
  line L8621 (100.304, -70.7141) -> (100.481, -70.7689)
  line L8622 (101.063, -71.6712) -> (101.039, -71.8551)
  line L8623 (234.248, -70.7347) -> (234.433, -70.7541)
  line L8624 (235.018, -72.2323) -> (234.897, -72.3727)
  line L8625 (233.292, -71.6715) -> (233.312, -71.4872)
  line L8626 (158.512, -73.14) -> (158.419, -73.1342)
  line L8627 (100.278, -72.5802) -> (100.093, -72.5944)
  line L8628 (99.7326, -72.5152) -> (99.5708, -72.4247)
  line L8629 (99.2297, -71.9944) -> (99.1786, -71.8161)
  line L8630 (234.773, -70.8971) -> (234.916, -71.0153)
  line L8631 (157.861, -72.7616) -> (157.793, -72.6018)
  line L8632 (99.4296, -72.3046) -> (99.3144, -72.1593)
  line L8633 (99.909, -72.5725) -> (99.7326, -72.5152)
  line L8634 (99.4483, -70.9659) -> (99.5928, -70.8497)
  line L8635 (-41.8657, -70.0968) -> (-41.6886, -70.1516)
  line L8636 (99.3144, -72.1593) -> (99.2297, -71.9944)
  line L8637 (100.457, -72.5304) -> (100.278, -72.5802)
  line L8638 (-41.3827, -70.358) -> (-41.2655, -70.5016)
  line L8639 (233.721, -70.8898) -> (233.886, -70.8039)
  line L8640 (-41.2655, -70.5016) -> (-41.1784, -70.6654)
  line L8641 (233.577, -71.006) -> (233.721, -70.8898)
  line L8642 (101.039, -71.8551) -> (100.981, -72.0311)
  line L8643 (-41.5255, -70.2398) -> (-41.3827, -70.358)
  line L8644 (233.358, -72.0344) -> (233.307, -71.8562)
  line L8645 (235.168, -71.8952) -> (235.109, -72.0711)
  line L8646 (234.038, -72.6126) -> (233.861, -72.5553)
  line L8647 (100.644, -70.8571) -> (100.787, -70.9753)
  line L8648 (-41.6886, -70.1516) -> (-41.5255, -70.2398)
  line L8649 (100.768, -72.3326) -> (100.622, -72.4468)
  line L8650 (-41.1249, -70.8428) -> (-41.1068, -71.0274)
  line L8651 (-41.1068, -71.0274) -> (-41.1071, -71.0539)
  line L8652 (100.787, -70.9753) -> (100.904, -71.1189)
  line L8653 (233.699, -72.4648) -> (233.558, -72.3446)
  line L8654 (100.481, -70.7689) -> (100.644, -70.8571)
  line L8655 (160.113, -72.8393) -> (159.993, -72.9654)
  line L8656 (101.045, -71.4601) -> (101.063, -71.6447)
  line L8657 (234.897, -72.3727) -> (234.751, -72.4868)
  line L8658 (159.512, -73.14) -> (158.512, -73.14)
  line L8659 (233.307, -71.8562) -> (233.292, -71.6715)
  line L8660 (100.991, -71.2826) -> (101.045, -71.4601)
  line L8661 (233.558, -72.3446) -> (233.443, -72.1993)
  line L8662 (235.109, -72.0711) -> (235.018, -72.2323)
  line L8663 (158.339, -71.6601) -> (158.512, -71.64)
  line L8664 (233.458, -71.148) -> (233.577, -71.006)
  line L8665 (234.222, -72.6345) -> (234.038, -72.6126)
  line L8666 (233.861, -72.5553) -> (233.699, -72.4648)
  line L8667 (233.443, -72.1993) -> (233.358, -72.0344)
  line L8668 (233.312, -71.4872) -> (233.368, -71.3105)
  line L8669 (157.963, -72.9015) -> (157.861, -72.7616)
  line L8670 (159.993, -72.9654) -> (159.848, -73.0606)
  line L8671 (157.911, -71.9407) -> (158.031, -71.8146)
  line L8672 (233.886, -70.8039) -> (234.064, -70.7515)
  line L8673 (100.904, -71.1189) -> (100.991, -71.2826)
  line L8674 (159.512, -71.64) -> (159.605, -71.6458)
  line L8675 (234.407, -72.6203) -> (234.222, -72.6345)
  line L8676 (233.368, -71.3105) -> (233.458, -71.148)
  line L8677 (234.585, -72.5704) -> (234.407, -72.6203)
  line L8678 (157.763, -72.4306) -> (157.774, -72.2572)
  line L8679 (235.12, -71.3227) -> (235.173, -71.5002)
  line L8680 (-42.9299, -70.6531) -> (-42.8406, -70.4906)
  line L8681 (-42.5769, -70.2324) -> (-42.4126, -70.1465)
  line L8682 (158.512, -69.1) -> (159.512, -69.1)
  line L8683 (157.861, -70.2216) -> (157.793, -70.0618)
  line L8684 (99.7571, -70.7638) -> (99.935, -70.7115)
  line L8685 (-41.1889, -71.4138) -> (-41.2805, -71.575)
  line L8686 (160.061, -69.3385) -> (160.163, -69.4784)
  line L8687 (176.403, -69.4784) -> (176.471, -69.6382)
  line L8688 (158.339, -69.1201) -> (158.512, -69.1)
  line L8689 (176.471, -69.6382) -> (176.501, -69.8094)
  line L8690 (159.773, -69.147) -> (159.928, -69.226)
  line L8691 (99.2398, -71.2704) -> (99.3291, -71.1079)
  line L8692 (176.501, -69.8094) -> (176.49, -69.9828)
  line L8693 (-42.4371, -71.8979) -> (-42.5989, -71.8075)
  line L8694 (159.848, -70.5206) -> (159.685, -70.5799)
  line L8695 (158.176, -69.1794) -> (158.339, -69.1201)
  line L8696 (160.25, -69.9828) -> (160.2, -70.1491)
  line L8697 (-43.0067, -71.0141) -> (-42.986, -70.8299)
  line L8698 (100.622, -72.4468) -> (100.457, -72.5304)
  line L8699 (159.512, -70.6) -> (158.512, -70.6)
  line L8700 (99.5928, -70.8497) -> (99.7571, -70.7638)
  line L8701 (-42.4126, -70.1465) -> (-42.2348, -70.0942)
  line L8702 (99.5708, -72.4247) -> (99.4296, -72.3046)
  line L8703 (-41.1071, -71.0539) -> (-41.1304, -71.2378)
  line L8704 (99.1837, -71.4471) -> (99.2398, -71.2704)
  line L8705 (99.1786, -71.8161) -> (99.1631, -71.6314)
  line L8706 (99.935, -70.7115) -> (100.12, -70.6947)
  line L8707 (-41.2805, -71.575) -> (-41.4016, -71.7153)
  line L8708 (-42.8406, -70.4906) -> (-42.7214, -70.3486)
  line L8709 (159.928, -69.226) -> (160.061, -69.3385)
  line L8710 (-41.7132, -71.9131) -> (-41.8918, -71.9629)
  line L8711 (100.093, -72.5944) -> (99.909, -72.5725)
  line L8712 (-42.9912, -71.1989) -> (-43.0067, -71.0141)
  line L8713 (-41.5477, -71.8295) -> (-41.7132, -71.9131)
  line L8714 (100.12, -70.6947) -> (100.304, -70.7141)
  line L8715 (-41.8918, -71.9629) -> (-42.0767, -71.9772)
  line L8716 (160.2, -70.1491) -> (160.113, -70.2993)
  line L8717 (-42.7401, -71.6873) -> (-42.8553, -71.542)
  line L8718 (99.1631, -71.6314) -> (99.1837, -71.4471)
  line L8719 (-42.5989, -71.8075) -> (-42.7401, -71.6873)
  line L8720 (160.231, -69.6382) -> (160.261, -69.8094)
  line L8721 (-42.7214, -70.3486) -> (-42.5769, -70.2324)
  line L8722 (-41.1304, -71.2378) -> (-41.1889, -71.4138)
  line L8723 (100.981, -72.0311) -> (100.889, -72.1923)
  line L8724 (-42.986, -70.8299) -> (-42.9299, -70.6531)
  line L8725 (160.113, -70.2993) -> (159.993, -70.4254)
  line L8726 (-41.4016, -71.7153) -> (-41.5477, -71.8295)
  line L8727 (-42.94, -71.3771) -> (-42.9912, -71.1989)
  line L8728 (160.163, -69.4784) -> (160.231, -69.6382)
  line L8729 (158.031, -69.2746) -> (158.176, -69.1794)
  line L8730 (-42.0501, -70.0774) -> (-41.8657, -70.0968)
  line L8731 (100.889, -72.1923) -> (100.768, -72.3326)
  line L8732 (-41.1784, -70.6654) -> (-41.1249, -70.8428)
  line L8733 (-42.2348, -70.0942) -> (-42.0501, -70.0774)
  line L8734 (176.013, -69.147) -> (176.168, -69.226)
  line L8735 (176.168, -69.226) -> (176.301, -69.3385)
  line L8736 (-42.0767, -71.9772) -> (-42.2608, -71.9552)
  line L8737 (157.911, -69.4007) -> (158.031, -69.2746)
  line L8738 (159.685, -70.5799) -> (159.512, -70.6)
  line L8739 (160.261, -69.8094) -> (160.25, -69.9828)
  line L8740 (99.3291, -71.1079) -> (99.4483, -70.9659)
  line L8741 (159.605, -69.1058) -> (159.773, -69.147)
  line L8742 (-42.8553, -71.542) -> (-42.94, -71.3771)
  line L8743 (-42.2608, -71.9552) -> (-42.4371, -71.8979)
  line L8744 (-54.7165, -66.9299) -> (-54.4919, -67.1013)
  line L8745 (175.752, -69.1) -> (175.845, -69.1058)
  line L8746 (-54.4919, -67.1013) -> (-54.2937, -67.3026)
  line L8747 (-55.5017, -66.6261) -> (-55.2264, -66.6899)
  line L8748 (174.014, -69.7172) -> (174.064, -69.5509)
  line L8749 (176.301, -69.3385) -> (176.403, -69.4784)
  line L8750 (158.419, -70.5942) -> (158.251, -70.553)
  line L8751 (158.251, -70.553) -> (158.096, -70.474)
  line L8752 (176.49, -69.9828) -> (176.44, -70.1491)
  line L8753 (-54.2937, -67.3026) -> (-54.1259, -67.5298)
  line L8754 (174.752, -70.6) -> (174.659, -70.5942)
  line L8755 (-53.9917, -67.7785) -> (-53.8939, -68.0435)
  line L8756 (174.491, -70.553) -> (174.336, -70.474)
  line L8757 (-53.8185, -68.7271) -> (-53.8561, -69.0071)
  line L8758 (174.336, -70.474) -> (174.203, -70.3615)
  line L8759 (-55.2264, -66.6899) -> (-54.963, -66.7918)
  line L8760 (-54.1259, -67.5298) -> (-53.9917, -67.7785)
  line L8761 (174.416, -69.1794) -> (174.579, -69.1201)
  line L8762 (174.151, -69.4007) -> (174.271, -69.2746)
  line L8763 (-56.7225, -70.3835) -> (-56.9645, -70.2378)
  line L8764 (-56.8595, -66.8962) -> (-56.6088, -66.766)
  line L8765 (-57.2938, -67.2555) -> (-57.0894, -67.0605)
  line L8766 (-55.3476, -70.5462) -> (-55.6263, -70.5926)
  line L8767 (-57.7166, -67.9835) -> (-57.6106, -67.7216)
  line L8768 (174.271, -69.2746) -> (174.416, -69.1794)
  line L8769 (157.763, -69.8906) -> (157.774, -69.7172)
  line L8770 (-54.963, -66.7918) -> (-54.7165, -66.9299)
  line L8771 (-56.4624, -70.4937) -> (-56.7225, -70.3835)
  line L8772 (-57.6106, -67.7216) -> (-57.4687, -67.4773)
  line L8773 (-54.5887, -70.1818) -> (-54.8236, -70.3388)
  line L8774 (176.088, -70.5206) -> (175.925, -70.5799)
  line L8775 (-56.6088, -66.766) -> (-56.3423, -66.6724)
  line L8776 (175.752, -70.6) -> (174.752, -70.6)
  line L8777 (-54.1965, -69.7771) -> (-54.3783, -69.9933)
  line L8778 (-56.3423, -66.6724) -> (-56.0652, -66.6173)
  line L8779 (-57.1836, -70.0594) -> (-57.3754, -69.852)
  line L8780 (174.579, -69.1201) -> (174.752, -69.1)
  line L8781 (175.845, -69.1058) -> (176.013, -69.147)
  line L8782 (-53.8145, -68.6015) -> (-53.8185, -68.7271)
  line L8783 (176.353, -70.2993) -> (176.233, -70.4254)
  line L8784 (157.963, -70.3615) -> (157.861, -70.2216)
  line L8785 (174.101, -70.2216) -> (174.033, -70.0618)
  line L8786 (174.003, -69.8906) -> (174.014, -69.7172)
  line L8787 (176.233, -70.4254) -> (176.088, -70.5206)
  line L8788 (-53.8939, -68.0435) -> (-53.8345, -68.3197)
  line L8789 (174.752, -69.1) -> (175.752, -69.1)
  line L8790 (159.512, -69.1) -> (159.605, -69.1058)
  line L8791 (-53.8345, -68.3197) -> (-53.8145, -68.6015)
  line L8792 (175.925, -70.5799) -> (175.752, -70.6)
  line L8793 (174.064, -69.5509) -> (174.151, -69.4007)
  line L8794 (174.203, -70.3615) -> (174.101, -70.2216)
  line L8795 (174.659, -70.5942) -> (174.491, -70.553)
  line L8796 (-54.8236, -70.3388) -> (-55.0783, -70.4611)
  line L8797 (176.44, -70.1491) -> (176.353, -70.2993)
  line L8798 (-57.6623, -69.3669) -> (-57.7517, -69.0989)
  line L8799 (174.033, -70.0618) -> (174.003, -69.8906)
  line L8800 (-56.9645, -70.2378) -> (-57.1836, -70.0594)
  line L8801 (-57.0894, -67.0605) -> (-56.8595, -66.8962)
  line L8802 (157.774, -69.7172) -> (157.824, -69.5509)
  line L8803 (157.824, -69.5509) -> (157.911, -69.4007)
  line L8804 (157.793, -70.0618) -> (157.763, -69.8906)
  line L8805 (159.993, -70.4254) -> (159.848, -70.5206)
  line L8806 (158.512, -70.6) -> (158.419, -70.5942)
  line L8807 (158.096, -70.474) -> (157.963, -70.3615)
  line L8808 (249.37, -67.9434) -> (249.22, -68.1832)